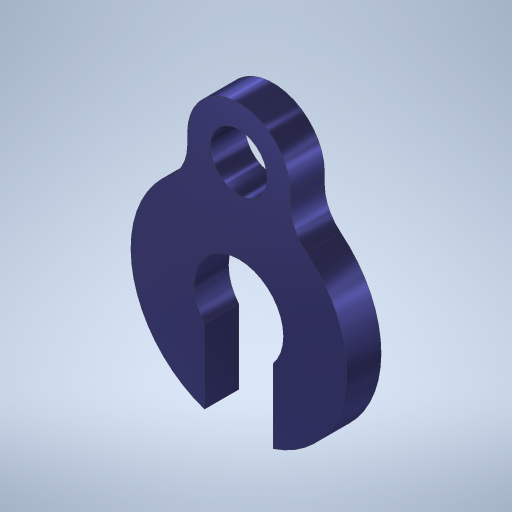
# Autodesk Inventor part: Front Suspension Adjustment Clip
Saved by Autodesk Inventor 2023.1 (Build 271208000, 208)
## iProperties
Created: 2019-11-22
Part Number: Front Suspension Adjustment Clip
Material: Generic
Document SubType Name: Modeling
Designer: Jopa
Density: 1 g/cm^3
Appearance: Poplar
Author: Jopa
Autodesk Inventor part; units mm, degrees
ref_plane "YZ Plane" through (0, 0, 0) normal (1, 0, 0) x (0, 1, 0)
ref_plane "XZ Plane" through (0, 0, 0) normal (0, 1, 0) x (-1, 0, 0)
ref_plane "XY Plane" through (0, 0, 0) normal (0, 0, 1) x (1, 0, 0)
sketch "Sketch1" plane through (0, 0, 0) normal (0, 0, 1) x (1, 0, 0)
  circle A0 centre (0, 0) radius 1.651 construction
  circle A1 centre (0, 4.7625) radius 1.0478
  arc A2 (1.905, 4.7625) -> (-1.905, 4.7625) centre (0, 4.7625) ccw
  line L0 (-1.905, 4.7625) -> (-1.905, 3.5178)
  line L1 (1.905, 4.7625) -> (1.905, 3.5178)
  arc A3 (-1.905, 3.5178) -> (-1.27, -3.7936) centre (0, 0) ccw
  line L2 (-1.27, -3.7936) -> (-1.27, -1.0549)
  line L3 (-6.0242, 0) -> (6.0242, 0) construction
  line L4 (0, -6.1357) -> (0, 8.8014) construction
  arc A4 (1.27, -3.7936) -> (1.905, 3.5178) centre (0, 0) ccw
  line L5 (1.27, -3.7936) -> (1.27, -1.0549)
  arc A5 (1.27, -1.0549) -> (-1.27, -1.0549) centre (0, 0) ccw
  dimension "d0" = 3.302
  dimension "d1" = 2.0955
  dimension "d2" = 4.7625
  dimension "d3" = 1.905
  dimension "d4" = 4.0005
  dimension "d5" = 2.54
  constraints: 8 end point, 8 point on circle, 5 centre point, 4 coincident, 3 vertical, 2 symmetric about line, 2 tangent, 1 horizontal alignment, 1 vertical alignment, 4 other
  measures "d1" diameter of A1
  measures "d2" distance of point (0, 0) A1.centre
  measures "d3" radius of A2
  measures "d4" radius of A3
  measures "d5" diameter of L2 L4
extrude "Extrusion1" add sketch "Sketch1" along normal mid plane 1.27
fillet "Fillet1" radius 1.5875 2 edges at (1.905, 3.5178, 0) (-1.905, 3.5178, 0)
body "Solid1"
